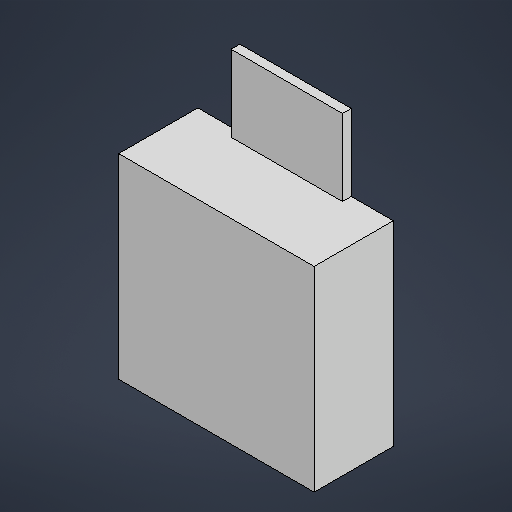
# Autodesk Inventor part: VLV101040A
Saved by Autodesk Inventor 2026 (Build 300175050, 175E)
## iProperties
Created: 2025-09-02
Part Number: VLV101040A
Material: 一般
Document SubType Name: Modeling
Designer: ka0n7
Density: 1 g/cm^3
Appearance: 既定
Author: ka0n7
Autodesk Inventor part; units mm, degrees
ref_plane "YZ Plane" through (0, 0, 0) normal (1, 0, 0) x (0, 1, 0)
ref_plane "XZ Plane" through (0, 0, 0) normal (0, 1, 0) x (-1, 0, 0)
ref_plane "XY Plane" through (0, 0, 0) normal (0, 0, 1) x (1, 0, 0)
sketch "スケッチ1" plane through (0, 0, 0) normal (0, 0, 1) x (1, 0, 0)
  line L0 (-5, -5) -> (5, -5)
  line L1 (5, -5) -> (5, 5)
  line L2 (5, 5) -> (-5, 5)
  line L3 (-5, 5) -> (-5, -5)
  line L4 (-5, -5) -> (5, 5) construction
  line L5 (5, -5) -> (-5, 5) construction
  point P0 (0, 0)
  dimension "d0" = 10
  dimension "d1" = 10
  constraints: 12 end point, 2 midpoint, 2 parallel, 1 horizontal, 1 perpendicular
  measures "d0" distance of L2.end L1.end
  measures "d1" distance of L0.end L1.end
extrude "押し出し1" add sketch "スケッチ1" along normal blind 4.05
sketch "スケッチ2" plane through (-5, 5, 0) normal (0, 1, 0) x (1, 0, 0)
  line L0 (5, 0) -> (2.15, 0)
  line L1 (10, 0) -> (0, 0) projected
  line L2 (2.15, 0) -> (7.85, 0)
  line L3 (7.85, 0) -> (7.85, -0.45)
  line L4 (7.85, -0.45) -> (2.15, -0.45)
  line L5 (2.15, -0.45) -> (2.15, 0)
  dimension "d4" = 2.85
  dimension "d5" = 5.7
  dimension "d6" = 0.45
  constraints: 10 end point, 2 parallel, 1 horizontal, 1 perpendicular, 1 point on line
  measures "d4" distance of L0.start L0.end
  measures "d5" distance of L3.end L4.end
  measures "d6" distance of L2.end L3.end
extrude "押し出し2" add sketch "スケッチ2" along normal blind 3.9
